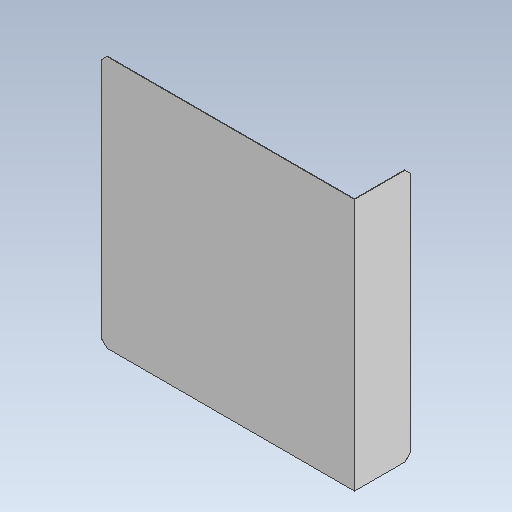
# Autodesk Inventor part: tag
Saved by Autodesk Inventor 2020 (Build 240168000, 168)
## iProperties
Created: 2022-07-09
Part Number: tag
Material: Generic
Document SubType Name: Modeling
Designer: Shuang Peng
Density: 1 g/cm^3
Appearance: Default
Author: Shuang Peng
Autodesk Inventor part; units mm, degrees
ref_plane "YZ Plane" through (0, 0, 0) normal (1, 0, 0) x (0, 1, 0)
ref_plane "XZ Plane" through (0, 0, 0) normal (0, 1, 0) x (-1, 0, 0)
ref_plane "XY Plane" through (0, 0, 0) normal (0, 0, 1) x (1, 0, 0)
sketch "Sketch1" plane through (0, 0, 0) normal (0, 0, 1) x (1, 0, 0)
  line L0 (22, -19) -> (22, 19) projected
  line L1 (-19, -22) -> (19, -22) projected
  line L2 (22.5, 22.5) -> (22.5, -22.5)
  line L3 (22.5, -22.5) -> (-22.5, -22.5)
  line L4 (-22.5, -22.5) -> (-22.5, 22.5)
  line L5 (-22.5, 22.5) -> (22.5, 22.5)
  line L6 (22.5, 22.5) -> (-22.5, -22.5) construction
  line L7 (22.5, -22.5) -> (-22.5, 22.5) construction
  point P0 (0, 0)
  dimension "d0" = 45
  dimension "d1" = 45
  constraints: 12 end point, 2 midpoint, 2 parallel, 2 perpendicular
  measures "d0" distance of L2.start L2.end
  measures "d1" distance of L2.end L3.end
extrude "Extrusion1" add sketch "Sketch1" along normal blind 0.1
sketch "Sketch2" plane through (22.5, -22.5, 0) normal (1, 0, 0) x (0, 0, -1)
  line L0 (-0.1, 0) -> (-0.1, 45) projected
  line L1 (0, 0) -> (0, 45) projected
  line L2 (0, 45) -> (-0.1, 45) projected
  line L3 (-0.1, 0) -> (-0.1, 45) projected
  line L4 (0, 0) -> (-0.1, 0) projected
  line L5 (-0.1, 0) -> (9.9, 0)
  line L6 (9.9, 0) -> (9.9, 45)
  line L7 (9.9, 45) -> (-0.1, 45)
  line L8 (-0.1, 45) -> (-0.1, 0)
  point P0 (0, 22.5)
  dimension "d4" = 10
  dimension "d5" = 45
  constraints: 8 end point, 2 parallel, 1 horizontal, 1 perpendicular
  measures "d4" distance of L7.end L6.end
  measures "d5" distance of L6.end L5.end
extrude "Extrusion2" add sketch "Sketch2" along normal blind 0.1
chamfer "Chamfer1" distance 1 angle 45 2 edges at (22.55, -22.5, -9.9) (22.55, 22.5, -9.9)
chamfer "Chamfer2" distance 1 angle 45 2 edges at (-22.5, 22.5, 0.05) (-22.5, -22.5, 0.05)
body "Solid1"
